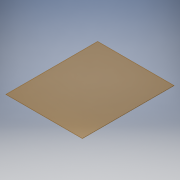
# Autodesk Inventor part: Floor
Saved by Autodesk Inventor 2016 SP1 (Build 200210100, 210)
## iProperties
Created: 2016-02-10
Part Number: Floor
Material: Polycarbonate, Smoke
Document SubType Name: Modeling
Designer: steele
Density: 1.2 g/cm^3
Appearance: Polycarbonate - Smoked
Author: steele
Autodesk Inventor part; units mm, degrees
ref_plane "YZ Plane" through (0, 0, 0) normal (1, 0, 0) x (0, 1, 0)
ref_plane "XZ Plane" through (0, 0, 0) normal (0, 1, 0) x (-1, 0, 0)
ref_plane "XY Plane" through (0, 0, 0) normal (0, 0, 1) x (1, 0, 0)
sketch "Sketch1" plane through (0, 0, 0) normal (0, 1, 0) x (-1, 0, 0)
  line L0 (635, 762) -> (-635, 762)
  line L1 (-635, 762) -> (-635, -762)
  line L2 (-635, -762) -> (635, -762)
  line L3 (635, -762) -> (635, 762)
  line L4 (635, 762) -> (-635, -762) construction
  line L5 (-635, 762) -> (635, -762) construction
  point P0 (0, 0)
  dimension "d0" = 1270
  dimension "d1" = 1524
  constraints: 12 end point, 2 midpoint, 2 parallel, 1 horizontal, 1 perpendicular
  measures "d0" distance of L0.start L0.end
  measures "d1" distance of L2.end L0.start
extrude "Extrusion1" add sketch "Sketch1" against normal blind 6.35
body "Solid1"
